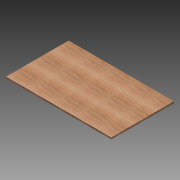
# Autodesk Inventor part: cart top
Saved by Autodesk Inventor 2013 (Build 170138000, 138)
## iProperties
Created: 2013-01-03
Part Number: cart top
Material: Wood (Birch)
Document SubType Name: Modeling
Designer: Arpan
Density: 1 g/cm^3
Author: Arpan
Autodesk Inventor part; units mm, degrees
ref_plane "YZ Plane" through (0, 0, 0) normal (1, 0, 0) x (0, 1, 0)
ref_plane "XZ Plane" through (0, 0, 0) normal (0, 1, 0) x (-1, 0, 0)
ref_plane "XY Plane" through (0, 0, 0) normal (0, 0, 1) x (1, 0, 0)
sketch "Sketch1" plane through (0, 0, 0) normal (0, 1, 0) x (-1, 0, 0)
  line L0 (-82.55, -82.55) -> (-1238.25, -82.55)
  line L1 (-1238.25, 603.25) -> (-82.55, 603.25)
  line L2 (-82.55, 603.25) -> (-82.55, -82.55)
  line L3 (-1238.25, -82.55) -> (-1238.25, 603.25)
  dimension "d20" = 685.8
  dimension "d21" = 1155.7
  constraints: 8 end point, 2 parallel, 1 horizontal, 1 perpendicular
  measures "d20" distance between parallel lines of L1 L0
  measures "d21" distance between parallel lines of L2 L3
extrude "Extrusion1" add sketch "Sketch1" along normal blind 19.05
body "Solid1"
